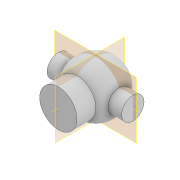
# Autodesk Inventor part: UpperlegY
Saved by Autodesk Inventor 2021 (Build 250183000, 183)
## iProperties
Created: 2020-12-19
Part Number: UpperlegY
Material: 一般
Document SubType Name: Modeling
Designer: Tazaki
Density: 2.06351 g/cm^3
Appearance: 既定
Mass: 500 g
Surface Area: 224.458 cm^2
Volume: 242.306 cm^3
Author: Tazaki
Autodesk Inventor part; units mm, degrees
ref_plane "XZ Plane" through (0, 0, 0) normal (0, 1, 0) x (-1, 0, 0)
sketch "スケッチ1" plane through (0, 0, 0) normal (0, 0, 1) x (1, 0, 0)
  arc A0 (0, 35) -> (0, -35) centre (0, 0) ccw
  line L0 (0, 35) -> (0, -35)
  dimension "d0" = 70
  constraints: 2 end point, 2 point on circle, 1 centre point, 1 coincident, 1 vertical
  measures "d0" diameter of A0
revolve "回転1" add sketch "スケッチ1" angle 360 about axis through (0, 35, 0) along (0, -1, 0)
sketch "スケッチ2" plane through (0, 0, 0) normal (0, 0, 1) x (1, 0, 0)
  circle A0 centre (0, 0) radius 25
  dimension "d2" = 50
  constraints: 1 centre point, 1 coincident
  measures "d2" diameter of A0
extrude "押し出し1" add sketch "スケッチ2" along normal blind 50
sketch "スケッチ3" plane through (0, 0, 0) normal (1, 0, 0) x (0, 1, 0)
  circle A0 centre (0, 0) radius 15
  dimension "d5" = 30
  constraints: 1 centre point, 1 coincident
  measures "d5" diameter of A0
extrude "押し出し2" add sketch "スケッチ3" along normal mid plane 100
